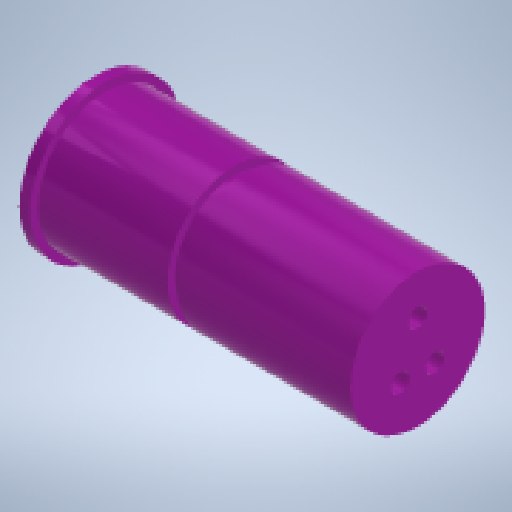
# Autodesk Inventor part: 028
Saved by Autodesk Inventor 2023 (Build 270158000, 158)
## iProperties
Created: 2022-04-04
Part Number: 028
Material: PC/ABS Plastic
Document SubType Name: Modeling
Designer: Vinicius Miguel
Density: 0.357273 g/cm^3
Appearance: Smooth - Purple
Mass: 6.10297 g
Surface Area: 114.249 cm^2
Volume: 17.0821 cm^3
Author: Vinicius Miguel
Autodesk Inventor part; units mm, degrees
ref_plane "YZ Plane" through (0, 0, 0) normal (1, 0, 0) x (0, 1, 0)
ref_plane "XZ Plane" through (0, 0, 0) normal (0, 1, 0) x (-1, 0, 0)
ref_plane "XY Plane" through (0, 0, 0) normal (0, 0, 1) x (1, 0, 0)
sketch "Sketch1" plane through (0, 0, 0) normal (0, 1, 0) x (-1, 0, 0)
  line L0 (0, 0) -> (55, 0)
  line L1 (55, 0) -> (55, -14)
  line L2 (55, -14) -> (53, -14)
  line L3 (53, -14) -> (53, -12.5)
  line L4 (53, -12.5) -> (0, -12.5)
  line L5 (0, -12.5) -> (0, 0)
  line L6 (55, 0) -> (65, 0)
  line L7 (65, 0) -> (65, -11)
  line L8 (65, -11) -> (55, -11)
  line L9 (5, 0) -> (5, -9.5)
  line L10 (5, -9.5) -> (65, -9.5)
  line L11 (32, -12.5) -> (32, -11)
  line L12 (32, -11) -> (34, -11)
  line L13 (34, -11) -> (34, -12.5)
  point P0 (55, -9.5)
  dimension "d0" = 25
  dimension "d1" = 28
  dimension "d2" = 2
  dimension "d3" = 55
  dimension "d5" = 10
  dimension "d6" = 5
  dimension "d7" = 3
  dimension "d17" = 22
  dimension "d18" = 2
  dimension "d19" = 32
  dimension "d20" = 22
  constraints: 28 end point, 11 perpendicular, 5 point on line, 2 horizontal, 1 vertical
  measures "d0" diameter of L4 L0
  measures "d1" diameter of L2 L0
  measures "d2" distance of L1.end L2.end
  measures "d3" distance of L0.start L0.end
  measures "d5" distance of L7.end L8.end
  measures "d6" distance between parallel lines of L5 L9
  measures "d7" distance between parallel lines of L4 L10
  measures "d17" diameter of L12 L0
  measures "d18" distance of L11.end L12.end
  measures "d19" distance from line of L11.start L5
  measures "d20" diameter of L8 L0
revolve "Revolution1" add sketch "Sketch1" angle 360 about axis through (0, 0, 0) along (-1, 0, 0) contours L0 L9 L10 L1 L2 L3 L4 L13 L12 L11 L5
sketch "Sketch2" plane through (0, 0, 0) normal (1, 0, 0) x (0, 0, -1)
  circle A0 centre (0, 0) radius 5
  line L0 (0, 0) -> (-5, 0)
  line L1 (0, 0) -> (-3.2139, -3.8302)
  point P0 (0, 5)
  point P1 (3.2139, -3.8302)
  dimension "d8" = 10
  dimension "d9" = 50
  constraints: 4 end point, 4 point on circle, 1 centre point, 1 coincident, 1 horizontal, 1 horizontal alignment, 1 vertical alignment
  measures "d8" diameter of A0
  measures "d9" angle of L0 L1
hole "Hole1" at (0, 5, 0) at (0, -3.8302, 3.2139) at (0, -3.8302, -3.2139) direction (-1, 0, 0) diameter 3.4 end through all clearance for "Countersunk Flat Head Screw ISO 2009/7046" size "M3" standard "ISO"
body "Solid1"
